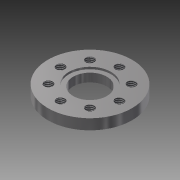
# Autodesk Inventor part: 3
Saved by Autodesk Inventor 2013 (Build 170138000, 138)
## iProperties
Created: 2014-02-07
Material: アルミニウム 6061
Document SubType Name: Modeling
Designer: andou
Density: 2.71 g/cm^3
Mass: 1.57929 g
Surface Area: 8.26239 cm^2
Volume: 0.582765 cm^3
Part Number: 3
Author: andou
Title: Bearing-Holder
Autodesk Inventor part; units mm, degrees
ref_plane "YZ Plane" through (0, 0, 0) normal (1, 0, 0) x (0, 1, 0)
ref_plane "XZ Plane" through (0, 0, 0) normal (0, 1, 0) x (-1, 0, 0)
ref_plane "XY Plane" through (0, 0, 0) normal (0, 0, 1) x (1, 0, 0)
sketch "スケッチ1" plane through (0, 0, 0) normal (0, 0, 1) x (1, 0, 0)
  circle A0 centre (0, 0) radius 10
  dimension "d0" = 20
  constraints: 1 centre point, 1 coincident
  measures "d0" diameter of A0
extrude "押し出し1" add sketch "スケッチ1" along normal blind 2.5
sketch "スケッチ2" plane through (0, 0, 2.5) normal (0, 0, 1) x (1, 0, 0)
  circle A0 centre (0, 0) radius 10 projected
  circle A1 centre (0, 0) radius 5
  dimension "d3" = 10
  constraints: 1 centre point, 1 coincident
  measures "d3" diameter of A1
hole "穴2" at (0, 0, 2.5) direction (0, 0, -1) diameter 10 depth 0.5
sketch "スケッチ4" plane through (0, 0, 2) normal (0, 0, 1) x (1, 0, 0)
  circle A0 centre (0, 0) radius 5 projected
  circle A1 centre (0, 0) radius 4
  dimension "d21" = 8
  constraints: 1 centre point, 1 coincident
  measures "d21" diameter of A1
hole "穴3" at (0, 0, 2) direction (0, 0, -1) diameter 8 end through all
sketch "スケッチ5" plane through (0, 0, 2.5) normal (0, 0, 1) x (1, 0, 0)
  circle A0 centre (0, 0) radius 5 projected
  circle A1 centre (0, 7) radius 1
  dimension "d29" = 7
  dimension "d30" = 2
  constraints: 1 centre point
  measures "d29" distance of A1.centre A0.centre
  measures "d30" diameter of A1
hole "穴4" at (0, 7, 2.5) direction (0, 0, -1) diameter 2 end through all
pattern_circular "円形状パターン1" count 8 over 360 about axis through (0, 0, 2.25) along (0, 0, 1) of "穴4"
thread "ねじ1" size "M2x0.4" class "6H" standard "ANSI Metric M Profile" full length
thread "ねじ2" size "M2x0.4" class "6H" standard "ANSI Metric M Profile" full length
thread "ねじ3" size "M2x0.4" class "6H" standard "ANSI Metric M Profile" full length
thread "ねじ4" size "M2x0.4" class "6H" standard "ANSI Metric M Profile" full length
thread "ねじ5" size "M2x0.4" class "6H" standard "ANSI Metric M Profile" full length
thread "ねじ6" size "M2x0.4" class "6H" standard "ANSI Metric M Profile" full length
thread "ねじ7" size "M2x0.4" class "6H" standard "ANSI Metric M Profile" full length
thread "ねじ8" size "M2x0.4" class "6H" standard "ANSI Metric M Profile" full length
